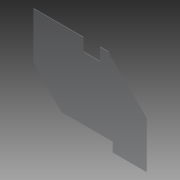
# Autodesk Inventor part: pneumatics board 1
Saved by Autodesk Inventor 2014 (Build 180170000, 170)
## iProperties
Created: 2014-01-20
Part Number: pneumatics board 1
Material: Polycarbonate, Clear
Document SubType Name: Modeling
Designer: Arpan
Density: 1.2 g/cm^3
Appearance: Polycarbonate - Clear
Author: Arpan
Autodesk Inventor part; units mm, degrees
ref_plane "YZ Plane" through (0, 0, 0) normal (1, 0, 0) x (0, 1, 0)
ref_plane "XZ Plane" through (0, 0, 0) normal (0, 1, 0) x (-1, 0, 0)
ref_plane "XY Plane" through (0, 0, 0) normal (0, 0, 1) x (1, 0, 0)
sketch "Sketch1" plane through (0, 0, 0) normal (0, 0, 1) x (1, 0, 0)
  line L0 (0, 0) -> (-150.114, 0)
  line L1 (1.016, 228.6) -> (1.016, 190.5)
  line L2 (1.016, 228.6) -> (-150.114, 228.6)
  line L3 (-150.114, 228.6) -> (-150.114, 0)
  line L4 (1.016, 190.5) -> (51.816, 190.5)
  line L5 (51.816, 190.5) -> (51.816, 228.6)
  line L6 (51.816, 228.6) -> (191.516, 228.6)
  line L7 (191.516, 228.6) -> (191.516, -28.575)
  line L8 (191.516, -28.575) -> (172.466, -28.575)
  line L9 (172.466, -28.575) -> (172.466, 0)
  line L10 (172.466, 0) -> (0, 0)
  dimension "d8" = 150.114
  dimension "d28" = 228.6
  dimension "d29" = 50.8
  dimension "d30" = 139.7
  dimension "d31" = 257.175
  dimension "d32" = 19.05
  dimension "d33" = 151.13
  dimension "d34" = 38.1
  constraints: 22 end point, 5 parallel, 4 perpendicular, 1 collinear, 1 horizontal
  measures "d8" distance of L0.start L0.end
  measures "d28" distance between parallel lines of L0 L2
  measures "d29" distance of L1.end L4.end
  measures "d30" distance of L5.end L6.end
  measures "d31" distance of L6.end L7.end
  measures "d32" distance of L7.end L8.end
  measures "d33" distance between parallel lines of L3 L1
  measures "d34" distance between parallel lines of L6 L4
extrude "Extrusion1" add sketch "Sketch1" along normal blind 1.5875
body "Solid1"
